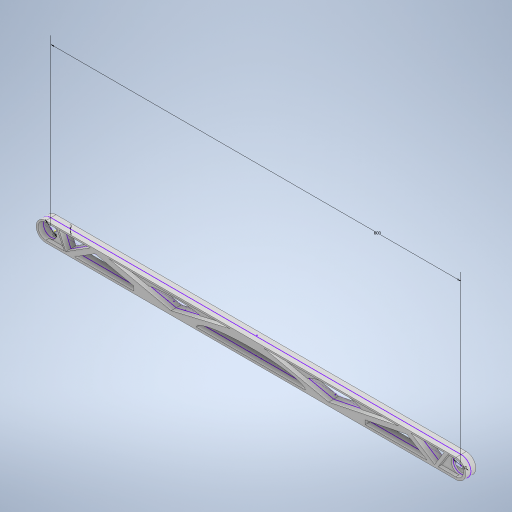
# Autodesk Inventor part: 05-15-2023 biella
Saved by Autodesk Inventor 2023 (Build 270158000, 158)
## iProperties
Created: 2023-05-12
Part Number: 05-15-2023 biella
Material: Generico
Document SubType Name: Modeling
Designer: Admin
Mass: 372.567 g
Surface Area: 1290.49 cm^2
Volume: 372.567 cm^3
Density: 1 g/cm^3
Appearance: Default
Author: Admin
Autodesk Inventor part; units mm, degrees
ref_plane "YZ Plane" through (0, 0, 0) normal (1, 0, 0) x (0, 1, 0)
ref_plane "XZ Plane" through (0, 0, 0) normal (0, 1, 0) x (-1, 0, 0)
ref_plane "XY Plane" through (0, 0, 0) normal (0, 0, 1) x (1, 0, 0)
sketch "Schizzo1" plane through (0, 0, 0) normal (0, 0, 1) x (1, 0, 0)
  circle A0 centre (-8.017891, 0.773321) radius 15
  circle A1 centre (791.982109, 0.773321) radius 15
  line L0 (-26.995892, 0) -> (811.346231, 0) construction
  line L1 (-8.222571, -18.773321) -> (792.57291, -18.773321)
  line L2 (792.57291, 18.773321) -> (-8.222571, 18.773321)
  arc A2 (-8.222571, 18.773321) -> (-8.222571, -18.773321) centre (-8.222571, 0) ccw
  arc A3 (792.57291, -18.773321) -> (792.57291, 18.773321) centre (792.57291, 0) ccw
  line L3 (-8.222571, 15.773321) -> (792.57291, 15.773321)
  line L4 (792.57291, -14.226679) -> (-8.222571, -14.226679)
  line L5 (350.886312, 15.773321) -> (236.489655, -11.192293)
  line L6 (543.983093, -11.979975) -> (417.954305, 15.773321)
  line L7 (236.489655, -11.192293) -> (114.812032, 15.773321)
  line L8 (201.054006, -14.226679) -> (87.83103, 10.865256)
  line L9 (680.037085, 15.773321) -> (543.983093, -11.979975)
  line L10 (697.011009, 10.048535) -> (577.160765, -14.226679)
  line L11 (13.627725, 15.773321) -> (27.70448, -14.226679)
  line L12 (17.741413, 15.773321) -> (30.638383, -14.226679)
  line L13 (30.638383, -14.226679) -> (78.112574, 15.773321)
  line L14 (87.83103, 10.865256) -> (48.123719, -14.226679)
  line L15 (776.982109, 15.773321) -> (758.215442, -14.226679)
  line L16 (769.519172, 15.773321) -> (750.752505, -14.226679)
  line L17 (750.752505, -14.226679) -> (705.029943, 15.773321)
  line L18 (697.011009, 10.048535) -> (735.816858, -14.226679)
  ellipse E0 centre (547.364845, -2.758251) end of major axis (495.28627, -2.758251) minor radius 12.662421 (598.813785, -0.795206) -> (495.618853, -1.329495) ccw
  ellipse E1 centre (232.342061, -2.399698) end of major axis (178.578758, -3.239205) minor radius 7.889612 (284.724407, 0.177617) -> (184.234682, 0.388205) ccw
  ellipse E2 centre (392.17517, -14.226679) end of major axis (286.104687, -14.226679) minor radius 18.338434 (498.245652, -14.226679) -> (286.104687, -14.226679) ccw
  arc A4 (163.415298, -5.885368) -> (163.227601, -14.226679) centre (182.513517, -10.487886) ccw
  arc A5 (615.828929, -14.226679) -> (615.059349, -6.550464) centre (577.160765, -14.226679) ccw
  point P0 (0, 0)
  point P1 (392.17517, 0)
  point P2 (256.078147, -14.226679)
  point P3 (528.138118, -14.226679)
  point P4 (394.110828, 21.023987)
  point P5 (-8.017891, -14.226679)
  point P6 (-8.017891, 15.773321)
  point P7 (791.982109, 15.773321)
  point P8 (791.982109, -14.226679)
  point P9 (219.889926, -7.51354)
  point P10 (249.388619, 15.773321)
  point P11 (254.036051, -7.056251)
  point P12 (379.733929, -14.226679)
  point P13 (402.890578, -14.226679)
  point P14 (417.954305, 15.773321)
  dimension "d0" = 30
  dimension "d1" = 30
  dimension "d2" = 800
  dimension "d3" = 3
  constraints: 36 end point, 10 point on circle, 10 point on line, 6 centre point, 4 tangent, 3 parallel, 1 coincident, 1 midpoint, 1 perpendicular, 49 other
  measures "d0" diameter of A0
  measures "d1" diameter of A1
  measures "d2" distance of A1.centre A0.centre
sketch "Schizzo1 outline for Estrusione9" plane through (0, 0, 0) normal (0, 0, 1) x (1, 0, 0)
  line L0 (-8.222571, -18.773321) -> (792.57291, -18.773321)
  arc A0 (-8.222571, 18.773321) -> (-8.222571, -18.773321) centre (-8.222571, 0) ccw
  arc A1 (792.57291, -18.773321) -> (792.57291, 18.773321) centre (792.57291, 0) ccw
  line L1 (792.57291, 18.773321) -> (-8.222571, 18.773321)
  line L2 (27.70448, -14.226679) -> (-8.017891, -14.226679)
  line L3 (13.627725, 15.773321) -> (27.70448, -14.226679)
  line L4 (-8.017891, 15.773321) -> (13.627725, 15.773321)
  arc A2 (-8.017891, -14.226679) -> (-8.017891, 15.773321) centre (-8.017891, 0.773321) cw
  line L5 (30.638383, -14.226679) -> (17.741413, 15.773321)
  line L6 (78.112574, 15.773321) -> (30.638383, -14.226679)
  line L7 (17.741413, 15.773321) -> (78.112574, 15.773321)
  line L8 (48.123719, -14.226679) -> (87.83103, 10.865256)
  line L9 (201.054006, -14.226679) -> (48.123719, -14.226679)
  line L10 (87.83103, 10.865256) -> (201.054006, -14.226679)
  line L11 (577.160765, -14.226679) -> (697.011009, 10.048535)
  line L12 (735.816858, -14.226679) -> (577.160765, -14.226679)
  line L13 (697.011009, 10.048535) -> (735.816858, -14.226679)
  line L14 (750.752505, -14.226679) -> (705.029943, 15.773321)
  line L15 (769.519172, 15.773321) -> (750.752505, -14.226679)
  line L16 (705.029943, 15.773321) -> (769.519172, 15.773321)
  line L17 (758.215442, -14.226679) -> (776.982109, 15.773321)
  line L18 (791.982109, -14.226679) -> (758.215442, -14.226679)
  arc A3 (791.982109, 15.773321) -> (791.982109, -14.226679) centre (791.982109, 0.773321) cw
  line L19 (776.982109, 15.773321) -> (791.982109, 15.773321)
extrude "Estrusione9" add sketch "Schizzo1 outline for Estrusione9" along normal mid plane 20
sketch "Schizzo1 outline for Estrusione10" plane through (0, 0, 0) normal (0, 0, 1) x (1, 0, 0)
  line L0 (87.83103, 10.865256) -> (48.123719, -14.226679)
  line L1 (201.054006, -14.226679) -> (87.83103, 10.865256)
  line L2 (48.123719, -14.226679) -> (201.054006, -14.226679)
  line L3 (30.638383, -14.226679) -> (78.112574, 15.773321)
  line L4 (17.741413, 15.773321) -> (30.638383, -14.226679)
  line L5 (78.112574, 15.773321) -> (17.741413, 15.773321)
  line L6 (705.029943, 15.773321) -> (750.752505, -14.226679)
  line L7 (769.519172, 15.773321) -> (705.029943, 15.773321)
  line L8 (750.752505, -14.226679) -> (769.519172, 15.773321)
  line L9 (735.816858, -14.226679) -> (697.011009, 10.048535)
  line L10 (577.160765, -14.226679) -> (735.816858, -14.226679)
  line L11 (697.011009, 10.048535) -> (577.160765, -14.226679)
  line L12 (417.954305, 15.773321) -> (543.983093, -11.979975)
  line L13 (680.037085, 15.773321) -> (417.954305, 15.773321)
  line L14 (543.983093, -11.979975) -> (680.037085, 15.773321)
  line L15 (114.812032, 15.773321) -> (236.489655, -11.192293)
  line L16 (350.886312, 15.773321) -> (114.812032, 15.773321)
  line L17 (236.489655, -11.192293) -> (350.886312, 15.773321)
extrude "Estrusione10" cut sketch "Schizzo1 outline for Estrusione10" along normal mid plane 4
extrude "Estrusione11" cut sketch "Schizzo1" along normal mid plane 20 contours L9 E0 L6 L3 | L9 L6 E0 | L5 E1 L7 L3 | L5 L7 E1
extrude "Estrusione12" add sketch "Schizzo1" along normal mid plane 7 contours L5 E1 L7 L3 | L5 L7 E1
extrude "Estrusione14" add sketch "Schizzo1" along normal mid plane 20 contours L9 E0 L6 L3 | L9 L6 E0
sketch "Schizzo1 outline for Estrusione15" plane through (0, 0, 0) normal (0, 0, 1) x (1, 0, 0)
  line L0 (27.70448, -14.226679) -> (13.627725, 15.773321)
  line L1 (-8.017891, -14.226679) -> (27.70448, -14.226679)
  arc A0 (-8.017891, 15.773321) -> (-8.017891, -14.226679) centre (-8.017891, 0.773321) cw
  line L2 (13.627725, 15.773321) -> (-8.017891, 15.773321)
  line L3 (776.982109, 15.773321) -> (758.215442, -14.226679)
  line L4 (791.982109, 15.773321) -> (776.982109, 15.773321)
  arc A1 (791.982109, -14.226679) -> (791.982109, 15.773321) centre (791.982109, 0.773321) cw
  line L5 (758.215442, -14.226679) -> (791.982109, -14.226679)
extrude "Estrusione15" add sketch "Schizzo1 outline for Estrusione15" along normal mid plane 7
extrude "Estrusione16" cut sketch "Schizzo1" along normal mid plane 20 contours L16 L17 L3 | L9 E0 L6 L3 | L9 L6 E0 | L5 E1 L7 L3 | L5 L7 E1 | L13 L12 L3
sketch "Schizzo1 outline for Estrusione17" plane through (0, 0, 0) normal (0, 0, 1) x (1, 0, 0)
  line L0 (417.954305, 15.773321) -> (543.983093, -11.979975)
  line L1 (680.037085, 15.773321) -> (417.954305, 15.773321)
  line L2 (543.983093, -11.979975) -> (680.037085, 15.773321)
extrude "Estrusione17" cut sketch "Schizzo1 outline for Estrusione17" along normal mid plane 20
sketch "Schizzo1 outline for Estrusione18" plane through (0, 0, 0) normal (0, 0, 1) x (1, 0, 0)
  line L0 (417.954305, 15.773321) -> (543.983093, -11.979975)
  line L1 (680.037085, 15.773321) -> (417.954305, 15.773321)
  line L2 (543.983093, -11.979975) -> (680.037085, 15.773321)
extrude "Estrusione18" add sketch "Schizzo1 outline for Estrusione18" along normal mid plane 4
extrude "Estrusione20" cut sketch "Schizzo1" along normal mid plane 20 contours L9 E0 L6 L3 | L9 L6 E0
extrude "Estrusione21" add sketch "Schizzo1" along normal mid plane 4 contours L9 E0 L6 L3 | L9 L6 E0 | L5 E1 L7 L3
extrude "Estrusione22" cut sketch "Schizzo1" along normal mid plane 20 contours L4 E2
extrude "Estrusione24" add sketch "Schizzo1" along normal mid plane 20 contours L4 L10 A5 | L4 A4 L8
extrude "Estrusione25" cut sketch "Schizzo1" along normal mid plane 20 contours L9 L6 E0
